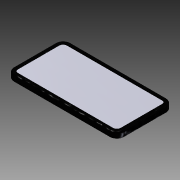
# Autodesk Inventor part: Phone
Saved by Autodesk Inventor 2014 SP1 (Build 180222100, 222)
## iProperties
Created: 2017-01-19
Part Number: Phone
Material: Generic
Document SubType Name: Modeling
Designer: danielsikar
Density: 1 g/cm^3
Appearance: Black
Author: danielsikar
Autodesk Inventor part; units mm, degrees
ref_plane "YZ Plane" through (0, 0, 0) normal (1, 0, 0) x (0, 1, 0)
ref_plane "XZ Plane" through (0, 0, 0) normal (0, 1, 0) x (-1, 0, 0)
ref_plane "XY Plane" through (0, 0, 0) normal (0, 0, 1) x (1, 0, 0)
sketch "Sketch1" plane through (0, 0, 0) normal (0, 0, 1) x (1, 0, 0)
  line L0 (0, 0) -> (142, 0)
  line L1 (142, 0) -> (142, 73)
  line L2 (142, 73) -> (0, 73)
  line L3 (0, 73) -> (0, 0)
  dimension "d0" = 142
  dimension "d1" = 73
  constraints: 8 end point, 2 parallel, 1 horizontal, 1 perpendicular
  measures "d0" distance of L2.end L1.end
  measures "d1" distance of L1.end L0.end
extrude "Extrusion1" add sketch "Sketch1" along normal blind 8.3
fillet "Fillet1" radius 10 4 edges at (142, 73, 4.15) (142, 0, 4.15) (0, 0, 4.15) (0, 73, 4.15)
fillet "Fillet2" radius 2 16 edges at (2.9289, 70.0711, 8.3) (0, 36.5, 8.3) (2.9289, 2.9289, 8.3) (71, 0, 8.3) (139.0711, 2.9289, 8.3) (142, 36.5, 8.3) (139.0711, 70.0711, 8.3) (71, 73, 8.3) (2.9289, 70.0711, 0) (0, 36.5, 0) (2.9289, 2.9289, 0) (71, 0, 0) (139.0711, 2.9289, 0) (142, 36.5, 0) (139.0711, 70.0711, 0) (71, 73, 0)
sketch "Sketch2" plane through (0, 0, 8.3) normal (0, 0, 1) x (1, 0, 0)
  arc A0 (10, 71) -> (2, 63) centre (10, 63) ccw projected
  line L0 (2, 10) -> (2, 63) projected
  arc A1 (2, 10) -> (10, 2) centre (10, 10) ccw projected
  line L1 (132, 2) -> (10, 2) projected
  arc A2 (132, 2) -> (140, 10) centre (132, 10) ccw projected
  line L2 (140, 63) -> (140, 10) projected
  arc A3 (140, 63) -> (132, 71) centre (132, 63) ccw projected
  line L3 (10, 71) -> (132, 71) projected
  arc A4 (136.9512, 63) -> (132, 67.9512) centre (132, 63) ccw
  line L4 (136.9512, 63) -> (136.9512, 10)
  arc A5 (132, 5.0488) -> (136.9512, 10) centre (132, 10) ccw
  line L5 (132, 5.0488) -> (10, 5.0488)
  arc A6 (5.0488, 10) -> (10, 5.0488) centre (10, 10) ccw
  line L6 (5.0488, 10) -> (5.0488, 63)
  arc A7 (10, 67.9512) -> (5.0488, 63) centre (10, 63) ccw
  line L7 (10, 67.9512) -> (132, 67.9512)
  point P0 (0, 0)
  constraints: 8 end point, 8 point on circle, 4 centre point, 7 other
extrude "Extrusion2" cut sketch "Sketch2" against normal blind 1 contours L4 A5 L5 A6 L6 A7 L7 A4
body "Solid1"
